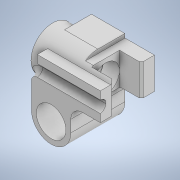
# Autodesk Inventor part: 411. Головка штока заднего хода
Saved by Autodesk Inventor 2021 (Build 250183000, 183)
## iProperties
Created: 2021-04-02
Part Number: 411. Головка штока заднего хода
Material: Типовые
Document SubType Name: Modeling
Designer: Данил
Density: 1 g/cm^3
Appearance: По умолчанию
Author: Данил
Autodesk Inventor part; units mm, degrees
ref_plane "YZ Plane" through (0, 0, 0) normal (1, 0, 0) x (0, 1, 0)
ref_plane "XZ Plane" through (0, 0, 0) normal (0, 1, 0) x (-1, 0, 0)
ref_plane "XY Plane" through (0, 0, 0) normal (0, 0, 1) x (1, 0, 0)
sketch "Эскиз3" plane through (0, 0, 0) normal (0, 0, 1) x (1, 0, 0)
  circle A0 centre (0, 0) radius 7.5
  circle A1 centre (0, 0) radius 10
  line L0 (-10, 0) -> (-10, 13)
  line L1 (-7, 16) -> (25, 16)
  line L2 (25, 16) -> (25, 12)
  line L3 (25, 12) -> (16, 12)
  arc A2 (-7, 16) -> (-10, 13) centre (-7, 13) ccw
  line L4 (10, 0) -> (10, 6)
  arc A3 (16, 12) -> (10, 6) centre (16, 6) ccw
  dimension "d15" = 15
  dimension "d16" = 20
  dimension "d17" = 3
  dimension "d18" = 4
  dimension "d19" = 6
  dimension "d20" = 35
  dimension "d21" = 16
  constraints: 10 end point, 6 point on circle, 4 centre point, 4 tangent, 3 vertical, 2 coincident, 2 horizontal alignment, 1 horizontal, 1 parallel
  measures "d15" diameter of A0
  measures "d16" diameter of A1
  measures "d17" radius of A2
  measures "d18" distance of L1.end L2.end
  measures "d19" radius of A3
  measures "d20" distance between parallel lines of L0 L2
  measures "d21" distance from line of L1 point (0, 0)
extrude "Выдавливание2" add sketch "Эскиз3" along normal mid plane 27.5
sketch "Эскиз6" plane through (0, 0, 0) normal (0, 0, 1) x (1, 0, 0)
  circle A0 centre (0, 0) radius 7.5 projected
  line L0 (-7.5, 0) -> (7.5, 0) construction
  line L1 (-14.4889, -3.8823) -> (14.4889, 3.8823)
  line L2 (14.4889, 3.8823) -> (15.1359, 1.4675)
  line L3 (15.1359, 1.4675) -> (-13.8418, -6.2971)
  line L4 (-13.8418, -6.2971) -> (-14.4889, -3.8823)
  line L5 (10, 6) -> (10, 0) projected
  arc A1 (-10, 0) -> (10, 0) centre (0, 0) ccw projected
  dimension "d31" = 15
  dimension "d32" = 5
  dimension "d33" = 30
  constraints: 10 end point, 3 perpendicular, 2 midpoint, 2 point on circle, 1 coincident, 1 horizontal
  measures "d31" angle of L0 L1
  measures "d32" diameter of L3 L1
  measures "d33" distance of L1.start L1.end
revolve "Вращение2" cut sketch "Эскиз6" angle 360 about axis through (-14.4889, -3.8823, 0) along (0.9659258, 0.258819, 0) contours A0 L3 L1 | A0 L1 L5 L3 | A0 L3 A1 L1 | L1 L2 L3 L5 | A1 L3 L4 L1
sketch "Эскиз7" plane through (0, 0, 0) normal (0, 0, 1) x (1, 0, 0)
  line L0 (25, 16) -> (-7, 16) projected
  line L1 (-7, 16) -> (25, 16) projected
  line L2 (-7, 16) -> (-7, 30)
  line L3 (-10, 0) -> (-10, 13) projected
  line L4 (-7, 30) -> (10, 30)
  line L5 (10, 30) -> (10, 28)
  line L6 (10, 28) -> (25, 28)
  line L7 (25, 16) -> (25, 12) projected
  line L8 (25, 28) -> (25, 16)
  line L9 (10, 6) -> (10, 0) projected
  line L10 (25, 12) -> (16, 12) projected
  point P0 (0, 0)
  point P1 (-7, 16)
  dimension "d35" = 3
  dimension "d36" = 30
  dimension "d37" = 16
  constraints: 10 end point, 4 perpendicular, 1 horizontal, 1 point on line, 1 vertical alignment
  measures "d35" distance between parallel lines of L3 L2
  measures "d36" distance from line of point (0, 0) L4
  measures "d37" distance between parallel lines of L10 L6
extrude "Выдавливание4" add sketch "Эскиз7" along normal mid plane 27.5
sketch "Эскиз8" plane through (0, 0, 0) normal (0, 0, 1) x (1, 0, 0)
  line L0 (-13, 19) -> (-7, 19)
  line L1 (-13, 30) -> (-7, 30)
  line L2 (-7, 30) -> (-7, 19)
  line L3 (-13, 30) -> (-13, 19)
  line L4 (-7, 16) -> (-7, 30) projected
  point P0 (0, 0)
  dimension "d40" = 19
  dimension "d41" = 22
  dimension "d42" = 6
  constraints: 9 end point, 2 horizontal, 1 coincident, 1 parallel, 1 perpendicular
  measures "d40" distance from line of point (0, 0) L0
  measures "d41" diameter of L1 L0
  measures "d42" distance of L1.start L1.end
revolve "Вращение3" add sketch "Эскиз8" angle 360 about axis through (-13, 19, 0) along (1, 0, 0)
fillet "Сопряжение1" radius 3 3 edges at (-9.066, 15.1752, -10.3136) (-9.066, 15.1752, 10.3136) (-10, 8, 0)
sketch "Эскиз9" plane through (10, 28, 13.75) normal (0, 1, 0) x (1, 0, 0)
  line L0 (-23, 2.75) -> (-23, 24.75) projected
  line L1 (-23, 3.8114) -> (-23, 23.6886) projected
  line L2 (14, 20.75) -> (4, 20.75)
  line L3 (4, 20.75) -> (4, 6.75)
  line L4 (4, 6.75) -> (14, 6.75)
  line L5 (15, 0) -> (15, 27.5) projected
  line L6 (15, 21.75) -> (15, 27.5)
  line L7 (15, 0) -> (0, 0) projected
  line L8 (15, 5.75) -> (15, 0)
  line L9 (15, 21.75) -> (14, 20.75)
  line L10 (15, 5.75) -> (14, 6.75)
  line L11 (15, 21.75) -> (15, 5.75)
  point P0 (-10, 13.75)
  point P1 (-23, 13.75)
  point P2 (15, 20.75)
  point P3 (15, 6.75)
  point P4 (4, 13.75)
  point P5 (-23, 13.75)
  dimension "d45" = 11
  dimension "d46" = 14
  dimension "d47" = 1
  dimension "d48" = 45
  dimension "d49" = 1
  dimension "d50" = 45
  constraints: 16 end point, 4 point on line, 3 midpoint, 1 collinear, 1 horizontal, 1 horizontal alignment, 1 parallel, 1 perpendicular, 1 vertical, 1 vertical alignment
  measures "d45" distance of point (15, 20.75) L2.end
  measures "d46" distance of L2.end L3.end
  measures "d47" distance of L6.start point (15, 20.75)
  measures "d48" angle of L6 L9
  measures "d49" distance of L8.start point (15, 6.75)
  measures "d50" angle of L8 L10
extrude "Выдавливание5" cut sketch "Эскиз9" against normal through all both and the other way through all
sketch "Эскиз10" plane through (-7, 30, 0) normal (-1, 0, 0) x (0, 0, 1)
  spline S0 degree 4 poles (11, -11) (11, -11.1642) (11.012, -11.3288) (11.0361, -11.4922) (11.0982, -11.7706) (11.1307, -11.8868) (11.1694, -12.0011) (11.2468, -12.1948) (11.2826, -12.2752) (11.3216, -12.3542) (11.4666, -12.6212) (11.5878, -12.8012) (11.7259, -12.9686) (12.0142, -13.2568) (12.1612, -13.3808) (12.3182, -13.4917) (12.5505, -13.6277) (12.6188, -13.6647) (12.6884, -13.6992) (12.8573, -13.776) (12.9577, -13.8159) (13.0598, -13.8509) (13.2751, -13.9134) (13.3885, -13.9401) (13.5031, -13.9608) (13.6512, -13.9798) (13.6841, -13.9836) (13.717, -13.9868) (13.75, -13.9896) knots 0 0 0 0 0 0.148007 0.148007 0.148007 0.256095 0.256095 0.256095 0.33491 0.33491 0.33491 0.528168 0.528168 0.528168 0.699584 0.699584 0.699584 0.769119 0.769119 0.769119 0.865802 0.865802 0.865802 0.97023 0.97023 0.97023 1 1 1 1 1 projected
  line L0 (13.75, 0) -> (13.75, -13.9896) projected
  line L1 (0, 0) -> (13.75, 0) projected
  arc A0 (11, -11) -> (0, 0) centre (0, -11) ccw projected
  line L2 (13.75, 0) -> (13.75, -13.9896) projected
  line L3 (13.75, -4) -> (8.4853, -4)
  arc A1 (9.9386, -15.7143) -> (-9.9386, -15.7143) centre (0, -11) ccw projected
  arc A2 (-9.9386, -15.7143) -> (9.9386, -15.7143) centre (0, -11) ccw projected
  arc A3 (13.75, -8) -> (10.8284, -11.6813) centre (13.75, -11) ccw
  arc A4 (10.8284, -11.6813) -> (13.75, -14) centre (13.75, -11) ccw
  point P0 (0, -30)
  point P1 (13.75, -4)
  point P2 (10.9477, -9.9289)
  dimension "d55" = 7
  dimension "d56" = 3
  dimension "d57" = 3
  constraints: 5 point on circle, 4 point on line, 2 centre point, 2 end point, 1 concentric, 1 horizontal alignment, 1 perpendicular, 1 other
  measures "d55" distance from line of L3 A0.centre
  measures "d56" radius of A3
  measures "d57" radius of A4
extrude "Выдавливание6" cut sketch "Эскиз10" along normal through all both and the other way through all contours A0 L1 L0 L3
extrude "Выдавливание7" cut sketch "Эскиз10" against normal through all contours A0 A3 L0 S0
sketch "Эскиз11" plane through (0, 0, 0) normal (0, 0, 1) x (1, 0, 0)
  line L0 (-13, 19) -> (14, 19)
  line L1 (-13, 19) -> (-13, 9)
  line L2 (-13, 9) -> (5, 9)
  line L3 (-13, 14.2857) -> (-13, 30) projected
  line L4 (5, 9) -> (5, 11.2)
  line L5 (5.8, 12) -> (14, 12)
  line L6 (5.8, 12) -> (5, 11.2)
  line L7 (14, 11.6569) -> (14, 28) projected
  line L8 (14, 12) -> (14, 19)
  point P0 (0, 0)
  point P1 (5, 12)
  point P2 (16, 12)
  dimension "d62" = 19
  dimension "d63" = 20
  dimension "d64" = 18
  dimension "d65" = 0.8
  dimension "d66" = 45
  constraints: 15 end point, 5 point on line, 3 perpendicular, 2 vertical, 1 horizontal, 1 horizontal alignment
  measures "d62" distance from line of point (0, 0) L0
  measures "d63" diameter of L2 L0
  measures "d64" distance of L1.end L2.end
  measures "d65" distance of L5.start point (5, 12)
  measures "d66" angle of L5 L6
revolve "Вращение4" cut sketch "Эскиз11" angle 360 about axis through (-13, 19, 0) along (1, 0, 0)
thread "Резьба1" size "M20x1" class "6H" standard "ISO Metric profile" length 6 offset 12
equation "\"d49\" = d47"
equation "\"d50\" = d48"
